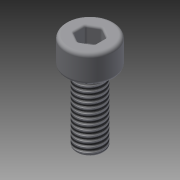
# Autodesk Inventor part: Cap(M4-10)
Saved by Autodesk Inventor 2013 (Build 170138000, 138)
## iProperties
Created: 2014-02-07
Material: 一般
Document SubType Name: Modeling
Designer: andou
Density: 1 g/cm^3
Author: andou
Title: Cap(M4-10)
Autodesk Inventor part; units mm, degrees
ref_plane "YZ Plane" through (0, 0, 0) normal (1, 0, 0) x (0, 1, 0)
ref_plane "XZ Plane" through (0, 0, 0) normal (0, 1, 0) x (-1, 0, 0)
ref_plane "XY Plane" through (0, 0, 0) normal (0, 0, 1) x (1, 0, 0)
sketch "スケッチ1" plane through (0, 0, 0) normal (0, 0, 1) x (1, 0, 0)
  circle A0 centre (0, 0) radius 3.5
  dimension "d0" = 7
  constraints: 1 centre point, 1 coincident
  measures "d0" diameter of A0
extrude "押し出し1" add sketch "スケッチ1" along normal blind 4
sketch "スケッチ2" plane through (0, 0, 0) normal (0, 0, -1) x (-1, 0, 0)
  circle A0 centre (0, 0) radius 3.5 projected
  circle A1 centre (0, 0) radius 2
  dimension "d3" = 4
  constraints: 1 centre point, 1 coincident
  measures "d3" diameter of A1
extrude "押し出し2" add sketch "スケッチ2" along normal blind 10 contours A1
sketch "スケッチ3" plane through (0, 0, 4) normal (0, 0, 1) x (1, 0, 0)
  circle A0 centre (0, 0) radius 3.5 projected
  line L0 (0, 1.7321) -> (1.5, 0.866)
  line L1 (1.5, 0.866) -> (1.5, -0.866)
  line L2 (1.5, -0.866) -> (0, -1.7321)
  line L3 (0, -1.7321) -> (-1.5, -0.866)
  line L4 (-1.5, -0.866) -> (-1.5, 0.866)
  line L5 (-1.5, 0.866) -> (0, 1.7321)
  dimension "d6" = 1.5
  constraints: 12 end point, 1 coincident, 13 other
  measures "d6" distance from line of point (0, 0) L0
extrude "押し出し3" cut sketch "スケッチ3" against normal blind 2.5 contours L0 L1 L2 L3 L4 L5
thread "ねじ1" size "M4x0.7" class "6g" standard "ANSI Metric M Profile" full length
fillet "フィレット1" radius 0.5 2 edges at (-3.5, 0, 4) (-3.5, 0, 0)
fillet "フィレット2" radius 0.3 19 edges at (-0.75, 1.299, 4) (-1.5, 0, 4) (-0.75, -1.299, 4) (0.75, -1.299, 4) (1.5, 0, 4) (0.75, 1.299, 4) (-0.75, 1.299, 1.5) (0.75, 1.299, 1.5) (0, 1.7321, 2.75) (-1.5, 0.866, 2.75) (-0.75, -1.299, 1.5) (-1.5, -0.866, 2.75) (-1.5, 0, 1.5) (1.5, 0, 1.5) (1.5, 0.866, 2.75) (1.5, -0.866, 2.75) (0.75, -1.299, 1.5) (0, -1.7321, 2.75) (2, 0, -10)
